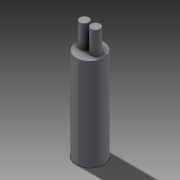
# Autodesk Inventor part: Part19
Saved by Autodesk Inventor 2014 (Build 180170000, 170)
## iProperties
Created: 2016-04-22
Part Number: Part19
Material: Stainless Steel
Document SubType Name: Modeling
Designer: admin
Density: 8.08 g/cm^3
Appearance: Semi-Polished
Author: admin
Autodesk Inventor part; units mm, degrees
ref_plane "YZ Plane" through (0, 0, 0) normal (1, 0, 0) x (0, 1, 0)
ref_plane "XZ Plane" through (0, 0, 0) normal (0, 1, 0) x (-1, 0, 0)
ref_plane "XY Plane" through (0, 0, 0) normal (0, 0, 1) x (1, 0, 0)
sketch "Sketch1" plane through (0, 0, 0) normal (0, 0, 1) x (1, 0, 0)
  circle A0 centre (0, 0) radius 3 projected
extrude "Extrusion1" add sketch "Sketch1" along normal blind 20
sketch "Sketch2" plane through (0, 0, 20) normal (0, 0, 1) x (1, 0, 0)
  circle A0 centre (0, 0) radius 3 projected
  circle A1 centre (-1.2, 0) radius 1
  circle A2 centre (1.2, 0) radius 1
  dimension "d2" = 2
  dimension "d3" = 2
  dimension "d4" = 1.2
  dimension "d5" = 1.2
  constraints: 2 centre point
  measures "d2" diameter of A1
  measures "d3" diameter of A2
  measures "d4" distance of A0.centre A1.centre
  measures "d5" distance of A0.centre A2.centre
extrude "Extrusion2" add sketch "Sketch2" along normal blind 5 separate body contours A1 | A2
body "Solid1"
body "Solid2"
